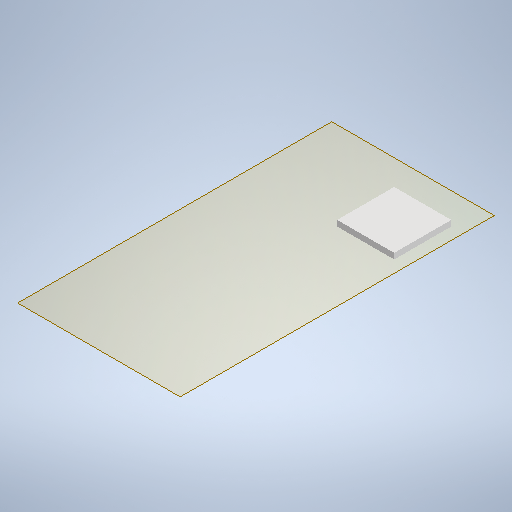
# Autodesk Inventor part: SIM7600G-H
Saved by Autodesk Inventor 2025.2 (Build 292293000, 293)
## iProperties
Created: 2025-06-06
Part Number: SIM7600G-H
Material: Generisch
Document SubType Name: Modeling
Designer: Jansc
Density: 1 g/cm^3
Appearance: Vorgabe
Author: Jansc
Autodesk Inventor part; units mm, degrees
ref_plane "YZ Plane" through (0, 0, 0) normal (1, 0, 0) x (0, 1, 0)
ref_plane "XZ Plane" through (0, 0, 0) normal (0, 1, 0) x (-1, 0, 0)
ref_plane "XY Plane" through (0, 0, 0) normal (0, 0, 1) x (1, 0, 0)
ref_plane "Arbeitsebene1" through (0, 0, 0) normal (0, 0, 1) x (1, 0, 0)
sketch "Skizze1" plane through (0, 0, 0) normal (0, 0, 1) x (1, 0, 0)
  line L0 (89.2067, -39.2918) -> (119.2067, -39.2918)
  line L1 (119.2067, -39.2918) -> (119.2067, -69.2918)
  line L2 (119.2067, -69.2918) -> (89.2067, -69.2918)
  line L3 (89.2067, -69.2918) -> (89.2067, -39.2918)
  point P0 (0, 0)
  dimension "d0" = 30
  dimension "d1" = 30
  constraints: 8 end point, 2 parallel, 1 horizontal, 1 perpendicular
  measures "d0" distance of L1.end L2.end
  measures "d1" distance of L0.end L1.end
extrude "Extrusion1" add sketch "Skizze1" along normal blind 3
